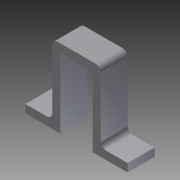
# Autodesk Inventor part: dudukan mini servo
Saved by Autodesk Inventor 2012 (Build 160160000, 160)
## iProperties
Created: 2013-01-07
Part Number: dudukan mini servo
Material: Default
Document SubType Name: Modeling
Designer: Irwan Haryanto
Density: 1 g/cm^3
Author: Irwan Haryanto
Autodesk Inventor part; units mm, degrees
ref_plane "YZ Plane" through (0, 0, 0) normal (1, 0, 0) x (0, 1, 0)
ref_plane "XZ Plane" through (0, 0, 0) normal (0, 1, 0) x (-1, 0, 0)
ref_plane "XY Plane" through (0, 0, 0) normal (0, 0, 1) x (1, 0, 0)
sketch "Sketch1" plane through (0, 0, 0) normal (0, 0, 1) x (1, 0, 0)
  line L0 (-9.0072, 10.9337) -> (2.9928, 10.9337)
  line L1 (2.9928, 10.9337) -> (2.9928, -15.0663)
  line L2 (-9.0072, -15.0663) -> (-9.0072, 10.9337)
  line L3 (-9.0072, -15.0663) -> (-22.0072, -15.0663)
  line L4 (2.9928, -15.0663) -> (15.9928, -15.0663)
  line L5 (15.9928, -12.0663) -> (7.9928, -12.0663)
  line L6 (5.9928, -10.0663) -> (5.9928, 11.9337)
  line L7 (3.9928, 13.9337) -> (-10.0072, 13.9337)
  line L8 (-12.0072, 11.9337) -> (-12.0072, -10.0663)
  line L9 (-14.0072, -12.0663) -> (-22.0072, -12.0663)
  line L10 (-22.0072, -15.0663) -> (-22.0072, -12.0663)
  line L11 (15.9928, -15.0663) -> (15.9928, -12.0663)
  arc A0 (-14.0072, -12.0663) -> (-12.0072, -10.0663) centre (-14.0072, -10.0663) ccw
  arc A1 (-10.0072, 13.9337) -> (-12.0072, 11.9337) centre (-10.0072, 11.9337) ccw
  arc A2 (5.9928, 11.9337) -> (3.9928, 13.9337) centre (3.9928, 11.9337) ccw
  arc A3 (5.9928, -10.0663) -> (7.9928, -12.0663) centre (7.9928, -10.0663) ccw
  point P0 (0, 0)
  point P1 (5.9928, -12.0663)
  point P2 (5.9928, 13.9337)
  point P3 (-12.0072, 13.9337)
  point P4 (-12.0072, -12.0663)
  dimension "d2" = 12
  dimension "d3" = 26
  dimension "d4" = 13
  dimension "d5" = 13
  dimension "d6" = 3
  dimension "d7" = 26
  dimension "d10" = 2
  dimension "d11" = 10
  constraints: 24 end point, 8 point on circle, 8 point on line, 8 tangent, 6 perpendicular, 4 centre point, 4 equal length, 3 equal radius, 1 horizontal, 2 other
  measures "d2" distance of L0.start L0.end
  measures "d3" distance of L0.end L1.end
  measures "d4" distance of L2.start L3.end
  measures "d5" distance of L1.end L4.end
  measures "d6" distance between parallel lines of L7 L0
  measures "d7" distance of L2.start L0.start
  measures "d10" radius of A0
  measures "d11" distance between parallel lines of L10 L8
extrude "Extrusion1" add sketch "Sketch1" along normal blind 10
body "Solid1"
